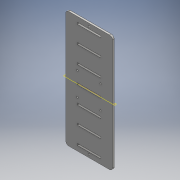
# Autodesk Inventor part: mounting_plate
Saved by Autodesk Inventor 2016 (Build 200138000, 138)
## iProperties
Created: 2018-10-08
Part Number: mounting_plate
Material: Generic
Document SubType Name: Modeling
Designer: andrew
Density: 1 g/cm^3
Appearance: Default
Author: andrew
Autodesk Inventor part; units mm, degrees
ref_plane "YZ Plane" through (0, 0, 0) normal (1, 0, 0) x (0, 1, 0)
ref_plane "XZ Plane" through (0, 0, 0) normal (0, 1, 0) x (-1, 0, 0)
ref_plane "XY Plane" through (0, 0, 0) normal (0, 0, 1) x (1, 0, 0)
sketch "Sketch1" plane through (0, 0, 0) normal (0, 1, 0) x (-1, 0, 0)
  line L0 (40, 100) -> (-40, 100)
  line L1 (-40, 100) -> (-40, -100)
  line L2 (-40, -100) -> (40, -100)
  line L3 (40, -100) -> (40, 100)
  line L4 (40, 100) -> (-40, -100) construction
  line L5 (-40, 100) -> (40, -100) construction
  point P0 (0, 0)
  dimension "d0" = 80
  dimension "d1" = 200
  constraints: 12 end point, 2 midpoint, 2 parallel, 1 horizontal, 1 perpendicular
  measures "d0" distance of L2.end L1.end
  measures "d1" distance of L1.end L0.end
extrude "Extrusion1" add sketch "Sketch1" along normal blind 3
sketch "Sketch2" plane through (0, 3, 0) normal (0, 1, 0) x (1, 0, 0)
  line L0 (-20, -20) -> (20, -20) construction
  line L1 (20, -20) -> (20, 20) construction
  line L2 (20, 20) -> (-20, 20) construction
  line L3 (-20, 20) -> (-20, -20) construction
  line L4 (-20, -20) -> (20, 20) construction
  line L5 (20, -20) -> (-20, 20) construction
  point P0 (0, 0)
  dimension "d4" = 40
  dimension "d5" = 40
  constraints: 12 end point, 4 coincident, 2 midpoint, 2 parallel, 1 horizontal, 1 perpendicular
  measures "d4" distance of L2.end L1.end
  measures "d5" distance of L1.end L0.end
hole "Hole1" at (-20, 3, 20) at (-20, 3, -20) at (20, 3, -20) at (20, 3, 20) direction (0, -1, 0) diameter 3 end through all
sketch "Sketch3" plane through (0, 3, 0) normal (0, 1, 0) x (1, 0, 0)
  line L0 (20, -1.5) -> (-20, -1.5)
  line L1 (-20, -1.5) -> (-20, 1.5)
  line L2 (-20, 1.5) -> (20, 1.5)
  line L3 (20, 1.5) -> (20, -1.5)
  line L4 (20, -1.5) -> (-20, 1.5) construction
  line L5 (-20, -1.5) -> (20, 1.5) construction
  line L6 (-20, -28.5) -> (20, -28.5)
  line L7 (-20, -31.5) -> (-20, -28.5)
  line L8 (20, -31.5) -> (-20, -31.5)
  line L9 (20, -28.5) -> (20, -31.5)
  line L10 (-20, -58.5) -> (20, -58.5)
  line L11 (-20, -61.5) -> (-20, -58.5)
  line L12 (20, -61.5) -> (-20, -61.5)
  line L13 (20, -58.5) -> (20, -61.5)
  line L14 (-20, -88.5) -> (20, -88.5)
  line L15 (-20, -91.5) -> (-20, -88.5)
  line L16 (20, -91.5) -> (-20, -91.5)
  line L17 (20, -88.5) -> (20, -91.5)
  line L18 (-20, 31.5) -> (20, 31.5)
  line L19 (-20, 28.5) -> (-20, 31.5)
  line L20 (20, 28.5) -> (-20, 28.5)
  line L21 (20, 31.5) -> (20, 28.5)
  line L22 (-20, 1.5) -> (20, 1.5)
  line L23 (-20, -1.5) -> (-20, 1.5)
  line L24 (20, -1.5) -> (-20, -1.5)
  line L25 (20, 1.5) -> (20, -1.5)
  line L26 (-20, -28.5) -> (20, -28.5)
  line L27 (-20, -31.5) -> (-20, -28.5)
  line L28 (20, -31.5) -> (-20, -31.5)
  line L29 (20, -28.5) -> (20, -31.5)
  line L30 (-20, -58.5) -> (20, -58.5)
  line L31 (-20, -61.5) -> (-20, -58.5)
  line L32 (20, -61.5) -> (-20, -61.5)
  line L33 (20, -58.5) -> (20, -61.5)
  line L34 (-20, 61.5) -> (20, 61.5)
  line L35 (-20, 58.5) -> (-20, 61.5)
  line L36 (20, 58.5) -> (-20, 58.5)
  line L37 (20, 61.5) -> (20, 58.5)
  line L38 (-20, 31.5) -> (20, 31.5)
  line L39 (-20, 28.5) -> (-20, 31.5)
  line L40 (20, 28.5) -> (-20, 28.5)
  line L41 (20, 31.5) -> (20, 28.5)
  line L42 (-20, 1.5) -> (20, 1.5)
  line L43 (-20, -1.5) -> (-20, 1.5)
  line L44 (20, -1.5) -> (-20, -1.5)
  line L45 (20, 1.5) -> (20, -1.5)
  line L46 (-20, -28.5) -> (20, -28.5)
  line L47 (-20, -31.5) -> (-20, -28.5)
  line L48 (20, -31.5) -> (-20, -31.5)
  line L49 (20, -28.5) -> (20, -31.5)
  line L50 (-20, 91.5) -> (20, 91.5)
  line L51 (-20, 88.5) -> (-20, 91.5)
  line L52 (20, 88.5) -> (-20, 88.5)
  line L53 (20, 91.5) -> (20, 88.5)
  line L54 (-20, 61.5) -> (20, 61.5)
  line L55 (-20, 58.5) -> (-20, 61.5)
  line L56 (20, 58.5) -> (-20, 58.5)
  line L57 (20, 61.5) -> (20, 58.5)
  line L58 (-20, 31.5) -> (20, 31.5)
  line L59 (-20, 28.5) -> (-20, 31.5)
  line L60 (20, 28.5) -> (-20, 28.5)
  line L61 (20, 31.5) -> (20, 28.5)
  line L62 (-20, 1.5) -> (20, 1.5)
  line L63 (-20, -1.5) -> (-20, 1.5)
  line L64 (20, -1.5) -> (-20, -1.5)
  line L65 (20, 1.5) -> (20, -1.5)
  point P0 (0, 0)
  dimension "d13" = 40
  dimension "d14" = 3
  dimension "d17" = 30
  dimension "d20" = 30
  constraints: 132 end point, 2 collinear, 2 midpoint, 2 parallel, 2 vertical, 1 horizontal, 1 perpendicular, 118 other
  measures "d13" distance of L1.end L2.end
  measures "d14" distance of L0.end L1.end
  measures "d17" distance of L1.end L6.start
  measures "d20" distance of L1.end L18.start
extrude "Extrusion2" cut sketch "Sketch3" against normal blind 3
sketch "Sketch4" plane through (0, 3, 0) normal (0, 1, 0) x (1, 0, 0)
  line L0 (-40, -100) -> (40, -100) construction
  line L1 (0, -100) -> (0, -95) construction
  point P0 (0, 0)
  dimension "d25" = 5
  constraints: 2 end point, 1 midpoint, 1 vertical
  measures "d25" distance of L1.start L1.end
hole "Hole2" at (0, 3, 95) direction (0, -1, 0) diameter 3 end through all
ref_plane "Work Plane1" through (-40, 0, 0) normal (0, 0, 1) x (1, 0, 0)
mirror "Mirror1" about plane through (-40, 0, 0) normal (0, 0, 1) of "Hole2"
fillet "Fillet1" radius 5 4 edges at (40, 1.5, 100) (-40, 1.5, 100) (40, 1.5, -100) (-40, 1.5, -100)
body "Solid1"
